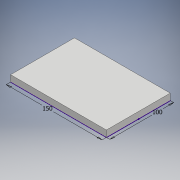
# Autodesk Inventor part: faceplate
Saved by Autodesk Inventor 2018 (Build 220112000, 112)
## iProperties
Created: 2019-06-23
Part Number: faceplate
Material: Generic
Document SubType Name: Modeling
Designer: ZEUSLAP
Density: 1 g/cm^3
Appearance: Default
Author: ZEUSLAP
Autodesk Inventor part; units mm, degrees
ref_plane "YZ Plane" through (0, 0, 0) normal (1, 0, 0) x (0, 1, 0)
ref_plane "XZ Plane" through (0, 0, 0) normal (0, 1, 0) x (-1, 0, 0)
ref_plane "XY Plane" through (0, 0, 0) normal (0, 0, 1) x (1, 0, 0)
sketch "Sketch1" plane through (0, 0, 0) normal (0, 0, 1) x (1, 0, 0)
  line L0 (-25.1368, 0) -> (22.6431, 0) construction
  line L1 (0, 13.6705) -> (0, -15.6298) construction
  line L2 (-75, 50) -> (75, 50)
  line L3 (75, 50) -> (75, -50)
  line L4 (75, -50) -> (-75, -50)
  line L5 (-75, -50) -> (-75, 50)
  point P0 (0, 0)
  point P1 (75, 0)
  point P2 (0, 50)
  dimension "d0" = 150
  dimension "d1" = 100
  constraints: 12 end point, 2 horizontal, 2 midpoint, 2 parallel, 1 horizontal alignment, 1 perpendicular, 1 vertical, 1 vertical alignment
  measures "d0" distance of L3.end L4.end
  measures "d1" distance of L2.end L3.end
extrude "Extrusion1" add sketch "Sketch1" along normal blind 10
body "Solid1"
